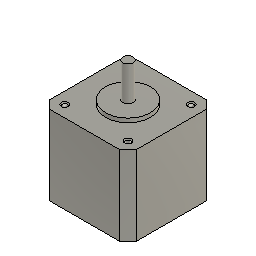
a2c38e86-3c35-49d0-80cf-e9d2caa12580 (Autodesk Fusion 360 design; units mm, degrees)
Autodesk Fusion 360 part; units mm, degrees
sketch "Sketch1" plane through (0, 0, 0) normal (0, 0, 1) x (1, 0, 0)
  line L0 (0, 0) -> (42.5, 0)
  line L1 (42.5, 0) -> (42.5, -42.5)
  line L2 (42.5, -42.5) -> (0, -42.5)
  line L3 (0, -42.5) -> (0, 0)
  dimension "d1" = 42.5
  dimension "d2" = 42.5
  constraint horizontal L0
  constraint vertical L1
  constraint horizontal L2
  constraint vertical L3
  constraint coincident L0.start L3.end
  measures "d1" distance of L0.start L0.end
  measures "d2" distance of L0.start L2.end
  measures "d14" diameter of L0.start
  measures "d17" diameter of L0.start
extrude "Extrude1" add sketch "Sketch1" against normal blind 39
sketch "Sketch2" plane through (0, 0, 0) normal (0, 0, 1) x (-1, 0, 0)
  line L0 (0, 42.5) -> (-42.5, 42.5)
  line L1 (-42.5, 42.5) -> (-42.5, 0)
  line L2 (-42.5, 0) -> (0, 0)
  line L3 (0, 0) -> (0, 42.5)
  line L4 (0, 0) -> (-42.5, 42.5)
  line L5 (-42.5, 0) -> (0, 42.5)
  line L6 (-5.75, 5.75) -> (-36.75, 5.75)
  line L7 (-36.75, 5.75) -> (-36.75, 36.75)
  line L8 (-36.75, 36.75) -> (-5.75, 36.75)
  line L9 (-5.75, 36.75) -> (-5.75, 5.75)
  circle A0 centre (-5.75, 5.75) radius 1.5
  circle A1 centre (-36.75, 5.75) radius 1.5
  circle A2 centre (-5.75, 36.75) radius 1.5
  circle A3 centre (-36.75, 36.75) radius 1.5
  dimension "d5" = 31
  dimension "d6" = 3
  dimension "d7" = 3
  dimension "d8" = 3
  dimension "d9" = 3
  constraint coincident L2.end L3.start
  constraint coincident L0.end L1.start
  constraint coincident L1.end L2.start
  constraint coincident L0.start L3.end
  constraint horizontal L6
  constraint vertical L7
  constraint horizontal L8
  constraint vertical L9
  constraint coincident L4 L7.end
  constraint coincident L4 L6.start
  constraint coincident L5 L6.end
  constraint coincident L6.start L9.end
  constraint coincident L6.end L7.start
  constraint coincident L8.end L9.start
  constraint coincident L7.end L8.start
  measures "d5" distance of L6.start L6.end
  measures "d6" diameter of A0
  measures "d7" diameter of A1
  measures "d8" diameter of A2
  measures "d9" diameter of A3
extrude "Extrude2" cut sketch "Sketch2" against normal blind 10 contours L5 L9 A2 | L5 L8 A2 | L4 L8 A3 | L4 L7 A3 | L4 L6 A0 | L4 L9 A0 | L5 L9 A2 | L5 L8 A2 | L5 L7 A1 | L5 L6 A1 | L4 L8 A3 | L4 L7 A3 | L4 L6 A0 | L4 L9 A0 | L5 L7 A1 | L5 L6 A1
chamfer "Chamfer1" distance 0.25 angle 45 4 edges at (7.1485, -6.2924, 0) (38.1485, -6.2924, 0) (38.1485, -37.2924, 0) (7.1485, -37.2924, 0)
thread "Thread1" "ISO Metric profile 3.0 M3x0.5 6H" major diameter 3.086 minor diameter 2.529 pitch 0.5 angle 60 resizes the face on face at (7.1322, -37.3327, -3.5) on face at (35.3678, -37.3327, -3.5) on face at (36.3437, -7.1939, -6.75) on face at (4.2575, -5.8994, -3.5)
chamfer "Chamfer2" distance 4 angle 45 4 edges at (42.5, 0, -19.5) (0, 0, -19.5) (0, -42.5, -19.5) (42.5, -42.5, -19.5)
sketch "Sketch3" plane through (0, 0, 0) normal (0, 0, 1) x (-1, 0, 0)
  circle A0 centre (-36.75, 36.75) radius 1.75
  circle A1 centre (-5.75, 5.75) radius 1.75
  line L0 (-38.5, 42.5) -> (-42.5, 38.5)
  line L1 (-42.5, 38.5) -> (-42.5, 4)
  line L2 (-42.5, 4) -> (-38.5, 0)
  line L3 (-38.5, 0) -> (-4, 0)
  line L4 (-4, 0) -> (0, 4)
  line L5 (0, 4) -> (0, 38.5)
  line L6 (0, 38.5) -> (-4, 42.5)
  line L7 (-4, 42.5) -> (-38.5, 42.5)
  circle A2 centre (-36.75, 5.75) radius 1.75
  circle A3 centre (-5.75, 36.75) radius 1.75
  line L8 (-5.75, 5.75) -> (-36.75, 36.75)
  line L9 (-36.75, 36.75) -> (-36.75, 5.75)
  line L10 (-36.75, 5.75) -> (-5.75, 36.75)
  circle A4 centre (-21.25, 21.25) radius 11
  dimension "d14" = 22
  constraint coincident A1.centre L8.start
  constraint coincident A0.centre L8.end
  constraint coincident A2.centre L9.end
  constraint coincident A3.centre L10.end
  constraint midpoint L10 A4.centre
  measures "d14" diameter of A4
extrude "Extrude3" add sketch "Sketch3" along normal blind 2 contours L8 L10 A4 | L8 L10 A4 | L8 L10 A4 | L8 L10 A4
sketch "Sketch4" plane through (0, 0, 2) normal (0, 0, 1) x (-1, 0, 0)
  circle A0 centre (-21.25, 21.25) radius 11
  circle A1 centre (-21.25, 21.25) radius 2.5
  dimension "d17" = 5
  constraint concentric A0 A1
  measures "d17" diameter of A1
extrude "Extrude4" add sketch "Sketch4" along normal blind 17 contours A1
